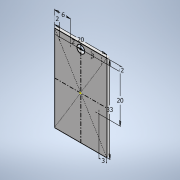
# Autodesk Inventor part: ShellyUni
Saved by Autodesk Inventor 2021 (Build 250183000, 183)
## iProperties
Created: 2021-04-10
Part Number: ShellyUni
Material: Generic
Document SubType Name: Modeling
Designer: James
Density: 1 g/cm^3
Appearance: Default
Author: James
Autodesk Inventor part; units mm, degrees
ref_plane "YZ Plane" through (0, 0, 0) normal (1, 0, 0) x (0, 1, 0)
ref_plane "XZ Plane" through (0, 0, 0) normal (0, 1, 0) x (-1, 0, 0)
ref_plane "XY Plane" through (0, 0, 0) normal (0, 0, 1) x (1, 0, 0)
sketch "Sketch1" plane through (0, 0, 0) normal (0, 0, 1) x (1, 0, 0)
  line L0 (-10, -16.5) -> (10, -16.5)
  line L1 (10, -16.5) -> (10, 16.5)
  line L2 (10, 16.5) -> (-10, 16.5)
  line L3 (-10, 16.5) -> (-10, -16.5)
  line L4 (-10, -16.5) -> (10, 16.5) construction
  line L5 (10, -16.5) -> (-10, 16.5) construction
  line L6 (0, 16.5) -> (0, -16.5)
  line L7 (-10, 0) -> (10, 0)
  circle A0 centre (0, 14.5) radius 1.5
  line L8 (-10, 14.5) -> (10, 14.5) construction
  line L9 (10, 14.5) -> (-10, 14.5) construction
  point P0 (0, 0)
  point P1 (-8, 14.5)
  point P2 (-4, 14.5)
  point P3 (8, 14.5)
  point P4 (4, 14.5)
  point P5 (7, -3.5)
  dimension "d0" = 20
  dimension "d1" = 33
  dimension "d2" = 3
  dimension "d3" = 2
  dimension "d4" = 2
  dimension "d5" = 6
  dimension "d6" = 2
  dimension "d7" = 20
  dimension "d8" = 3
  constraints: 20 end point, 6 midpoint, 6 point on line, 4 symmetric about line, 2 parallel, 2 perpendicular, 1 centre point, 1 horizontal
  measures "d0" distance of L2.end L1.end
  measures "d1" distance of L1.end L0.end
  measures "d2" diameter of A0
  measures "d3" distance from line of L2 A0.centre
  measures "d4" distance of L8.start point (-8, 14.5)
  measures "d5" distance from line of L3 point (-4, 14.5)
  measures "d6" distance between parallel lines of L2 L8
  measures "d7" distance from line of point (7, -3.5) L2
  measures "d8" distance from line of point (7, -3.5) L1
extrude "Extrusion1" add sketch "Sketch1" against normal blind 1
hole "Hole1" at (0, 14.5, 0) direction (0, 0, -1) diameter 3 end through all
body "Solid1"
